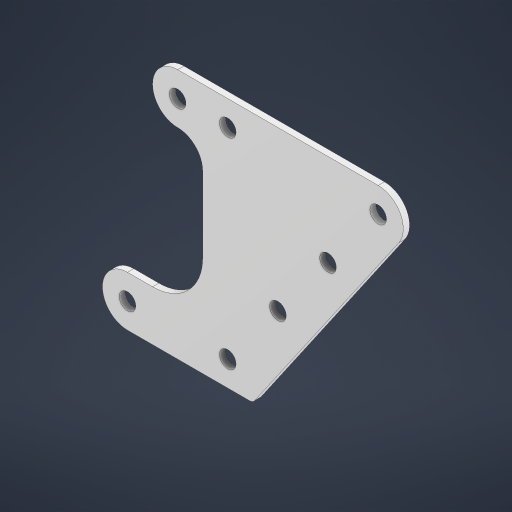
# Autodesk Inventor part: gusset
Saved by Autodesk Inventor 2024 (Build 280153000, 153)
## iProperties
Created: 2024-02-11
Part Number: gusset
Material: Acetal Resin, White
Document SubType Name: Modeling
Designer: Averey Ku
Density: 1.425 g/cm^3
Appearance: Smooth - White
d0: 0.165 in
d1: 0.165 in
d4: 0.063 in
d7: 0.250 in
d8: 0.500 in
d11: 0.165 in
d13: 0.165 in
Author: Averey Ku
Autodesk Inventor part; units mm, degrees
ref_plane "YZ Plane" through (0, 0, 0) normal (1, 0, 0) x (0, 1, 0)
ref_plane "XZ Plane" through (0, 0, 0) normal (0, 1, 0) x (-1, 0, 0)
ref_plane "XY Plane" through (0, 0, 0) normal (0, 0, 1) x (1, 0, 0)
sketch "main" plane through (0, 0, 0) normal (0, 0, 1) x (1, 0, 0)
  circle A0 centre (-11.3817, -22.2219) radius 2.0955
  circle A1 centre (-11.3817, 28.5781) radius 2.0955
  circle A2 centre (-24.0817, 28.5781) radius 2.0955
  arc A3 (-24.0817, 34.9281) -> (-24.0817, 22.2281) centre (-24.0817, 28.5781) ccw
  line L0 (-4.5584, -27.8865) -> (31.9434, 24.9697)
  line L1 (26.7183, 34.9281) -> (-24.0817, 34.9281)
  arc A4 (31.9434, 24.9697) -> (26.7183, 34.9281) centre (26.7183, 28.5781) ccw
  circle A5 centre (26.7183, 28.5781) radius 2.0955
  arc A6 (-5.8647, -28.5719) -> (-4.5584, -27.8865) centre (-5.8647, -26.9844) ccw
  line L2 (-36.7817, -15.8719) -> (-36.7817, -15.8719)
  line L3 (-36.7817, -28.5719) -> (-5.8647, -28.5719)
  circle A7 centre (-36.7817, -22.2219) radius 2.0955
  arc A8 (-36.7817, -15.8719) -> (-36.7817, -28.5719) centre (-36.7817, -22.2219) ccw
  line L4 (-17.7317, 15.8781) -> (-17.7317, -3.1719)
  line L5 (-30.4317, -15.8719) -> (-36.7817, -15.8719)
  line L6 (-24.0817, 22.2281) -> (-24.0817, 22.2281)
  arc A9 (-17.7317, 15.8781) -> (-24.0817, 22.2281) centre (-24.0817, 15.8781) ccw
  arc A10 (-30.4317, -15.8719) -> (-17.7317, -3.1719) centre (-30.4317, -3.1719) ccw
  circle A11 centre (1.3183, -5.2886) radius 2.0955
  circle A12 centre (14.0183, 11.6448) radius 2.0955
  point P0 (-15.5195, 2.5641)
  point P1 (-17.7317, 22.2281)
  dimension "d0" = 4.191
  dimension "d1" = 4.191
  dimension "d4" = 1.5875
  dimension "d7" = 6.35
  dimension "d8" = 12.7
  dimension "d11" = 4.191
  dimension "d13" = 4.191
  measures "d0" diameter of A0
  measures "d1" diameter of A1
  measures "d4" radius of A6
  measures "d7" radius of A9
  measures "d8" radius of A10
  measures "d11" diameter of A11
  measures "d13" diameter of A12
sketch "Sketch1" plane through (0, 0, 0) normal (0, 0, 1) x (1, 0, 0)
  circle A0 centre (25.4, 0) radius 2.0955
  circle A1 centre (25.4, 50.8) radius 2.0955
  circle A2 centre (12.7, 50.8) radius 2.0955
  arc A3 (12.7, 57.15) -> (12.7, 44.45) centre (12.7, 50.8) ccw
  line L0 (32.2233, -5.6646) -> (68.7251, 47.1916)
  line L1 (63.5, 57.15) -> (12.7, 57.15)
  arc A4 (68.7251, 47.1916) -> (63.5, 57.15) centre (63.5, 50.8) ccw
  circle A5 centre (63.5, 50.8) radius 2.0955
  arc A6 (30.917, -6.35) -> (32.2233, -5.6646) centre (30.917, -4.7625) ccw
  line L2 (0, 6.35) -> (0, 6.35)
  line L3 (0, -6.35) -> (30.917, -6.35)
  circle A7 centre (0, 0) radius 2.0955
  arc A8 (0, 6.35) -> (0, -6.35) centre (0, 0) ccw
  line L4 (19.05, 38.1) -> (19.05, 19.05)
  line L5 (6.35, 6.35) -> (0, 6.35)
  line L6 (12.7, 44.45) -> (12.7, 44.45)
  arc A9 (19.05, 38.1) -> (12.7, 44.45) centre (12.7, 38.1) ccw
  arc A10 (6.35, 6.35) -> (19.05, 19.05) centre (6.35, 19.05) ccw
  circle A11 centre (38.1, 16.9333) radius 2.0955
  circle A12 centre (50.8, 33.8667) radius 2.0955
  constraints: 1 other
extrude "Extrusion1" add sketch "Sketch1" along normal blind 1.5875
body "Solid1"
